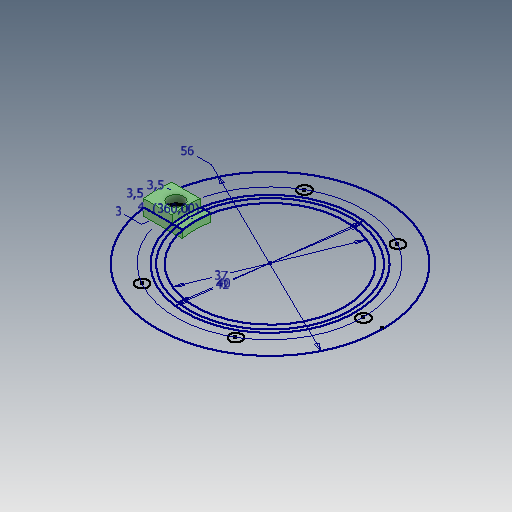
# Autodesk Inventor part: ClipsForLens
Saved by Autodesk Inventor 2020.3 (Build 243373000, 373)
## iProperties
Created: 2021-06-14
Part Number: ClipsForLens
Material: Generic
Document SubType Name: Modeling
Designer: Yusuf
Mass: 0.174287 g
Surface Area: 2.73488 cm^2
Volume: 0.174287 cm^3
Density: 1 g/cm^3
Appearance: Smooth - Dark Forest Green
Author: Yusuf
Autodesk Inventor part; units mm, degrees
ref_plane "YZ Plane" through (0, 0, 0) normal (1, 0, 0) x (0, 1, 0)
ref_plane "XZ Plane" through (0, 0, 0) normal (0, 1, 0) x (-1, 0, 0)
ref_plane "XY Plane" through (0, 0, 0) normal (0, 0, 1) x (1, 0, 0)
sketch "Sketch2" plane through (0, 0, 0) normal (0, 1, 0) x (-1, 0, 0)
  circle A0 centre (0, 0) radius 18.5
  circle A1 centre (0, 0) radius 28
  line L0 (18.5, 0) -> (28, 0) construction
  circle A2 centre (23.25, 0) radius 1.5
  circle A3 centre (11.625, 20.1351) radius 1.5
  circle A4 centre (-11.625, 20.1351) radius 1.5
  circle A5 centre (-23.25, 0) radius 1.5
  circle A6 centre (-11.625, -20.1351) radius 1.5
  circle A7 centre (11.625, -20.1351) radius 1.5
  circle A8 centre (0, 0) radius 20
  circle A9 centre (0, 0) radius 21
  line L1 (18.1659, 3.5) -> (27.7804, 3.5)
  line L2 (27.7804, -3.5) -> (18.1659, -3.5)
  circle A10 centre (23.25, 0) radius 2
  point P0 (-28, 0)
  point P1 (20.7063, -3.5)
  point P2 (20.7063, 3.5)
  dimension "d8" = 37
  dimension "d9" = 3
  dimension "d10" = 360
  dimension "d11" = 56
  dimension "d12" = 40
  dimension "d13" = 42
  dimension "d14" = 3.5
  dimension "d15" = 3.5
  dimension "d16" = 4
  constraints: 11 centre point, 6 coincident, 6 end point, 6 point on circle, 2 horizontal, 2 horizontal alignment, 1 midpoint, 1 parallel, 13 other
  measures "d8" diameter of A0
  measures "d9" diameter of A2
  measures "d11" diameter of A1
  measures "d12" diameter of A8
  measures "d13" diameter of A9
  measures "d14" distance between parallel lines of L0 L1
  measures "d15" distance between parallel lines of L0 L2
  measures "d16" diameter of A10
extrude "Extrusion1" add sketch "Sketch2" along normal blind 1.8 contours L1 A1 L2 A9 picked at (23.9926, 2.9951)
extrude "Extrusion2" add sketch "Sketch2" against normal blind 2 contours A0 L1 A8 L2 | L1 A9 L2 A8 | L1 A1 L2 A9 picked at (18.7362, 3.1137) picked at (20.0868, -3.1133) picked at (23.9926, 2.9951)
body "Solid1"
